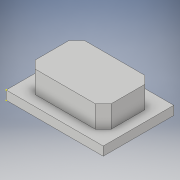
# Autodesk Inventor part: MiddleButton
Saved by Autodesk Inventor 2019 (Build 230136000, 136)
## iProperties
Created: 2021-04-22
Part Number: MiddleButton
Material: Všeobecné
Document SubType Name: Modeling
Designer: miko flosso
Density: 1 g/cm^3
Appearance: Výchozí
Author: miko flosso
Autodesk Inventor part; units mm, degrees
ref_plane "YZ Plane" through (0, 0, 0) normal (1, 0, 0) x (0, 1, 0)
ref_plane "XZ Plane" through (0, 0, 0) normal (0, 1, 0) x (-1, 0, 0)
ref_plane "XY Plane" through (0, 0, 0) normal (0, 0, 1) x (1, 0, 0)
sketch "Náčrt1" plane through (0, 0, 0) normal (0, 1, 0) x (-1, 0, 0)
  line L0 (0, 0) -> (-11, 0)
  line L1 (-11, 0) -> (-11, -8)
  line L2 (-11, -8) -> (0, -8)
  line L3 (0, -8) -> (0, 0)
  dimension "d0" = 11
  dimension "d1" = 8
  constraints: 8 end point, 2 parallel, 1 horizontal, 1 perpendicular
  measures "d0" distance of L2.end L1.end
  measures "d1" distance of L1.end L0.end
extrude "Vysunutí1" add sketch "Náčrt1" along normal blind 1
sketch "Náčrt2" plane through (0, 1, 0) normal (0, 1, 0) x (1, 0, 0)
  line L0 (1.2, 1.2) -> (9.8, 1.2)
  line L1 (9.8, 1.2) -> (9.8, 6.8)
  line L2 (9.8, 6.8) -> (1.2, 6.8)
  line L3 (1.2, 6.8) -> (1.2, 1.2)
  line L4 (11, 8) -> (0, 8) projected
  line L5 (0, 8) -> (0, 0) projected
  dimension "d4" = 8.6
  dimension "d5" = 5.6
  dimension "d6" = 1.2
  dimension "d7" = 1.2
  constraints: 8 end point, 2 parallel, 1 horizontal, 1 perpendicular
  measures "d4" distance of L2.end L1.end
  measures "d5" distance of L1.end L0.end
  measures "d6" distance between parallel lines of L2 L4
  measures "d7" distance between parallel lines of L5 L3
extrude "Vysunutí2" add sketch "Náčrt2" along normal blind 2.5
chamfer "Zkosení1" distance 0.9 angle 45 4 edges at (1.2, 2.25, -6.8) (1.2, 2.25, -1.2) (9.8, 2.25, -1.2) (9.8, 2.25, -6.8)
sketch "Náčrt3" plane through (0, 0, 0) normal (0, 0, 1) x (1, 0, 0)
  point P0 (0, 0)
sketch "Náčrt4" plane through (0, 1, 0) normal (0, 1, 0) x (1, 0, 0)
  point P0 (0, 0)
